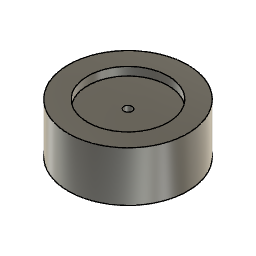
Roue v2 (Autodesk Fusion 360 design; units mm, degrees)
Autodesk Fusion 360 part; units mm, degrees
sketch "Esquisse1" plane through (0, 0, 0) normal (0, 0, 1) x (1, 0, 0)
  circle A0 centre (0, 0) radius 2.15
  dimension "d1" = 4.3
  constraint coincident A0.centre origin
  measures "d1" diameter of A0
extrude "Extrusion1" add sketch "Esquisse1" along normal blind 1.8
sketch "Esquisse2" plane through (0, 0, 1.8) normal (0, 0, 1) x (-1, 0, 0)
  circle A0 centre (0, 0) radius 2.15
  circle A1 centre (0, 0) radius 1.45
  dimension "d4" = 2.9
  constraint concentric A0 A1
  measures "d4" diameter of A1
extrude "Extrusion2" cut sketch "Esquisse2" against normal blind 0.3 contours A1
sketch "Esquisse3" plane through (0, 0, 0) normal (0, 0, -1) x (1, 0, 0)
  circle A0 centre (0, 0) radius 2.15
  circle A1 centre (0, 0) radius 1.1
  dimension "d7" = 2.2
  constraint concentric A0 A1
  measures "d7" diameter of A1
extrude "Extrusion3" cut sketch "Esquisse3" against normal blind 0.5 contours A1
sketch "Esquisse4" plane through (0, 0, 1.5) normal (0, 0, 1) x (-1, 0, 0)
  circle A0 centre (0, 0) radius 1.45
  circle A1 centre (0, 0) radius 0.15
  dimension "d10" = 0.3
  constraint concentric A0 A1
  measures "d10" diameter of A1
extrude "Extrusion4" cut sketch "Esquisse4" against normal blind 3.8 contours A1
scale "Echelle1" factor 10 about (1.45, 0, 1.8) bodies 1
